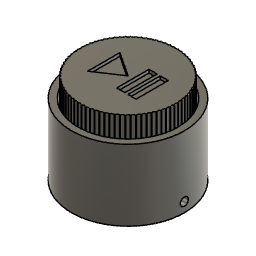
Volume knob v2 (Autodesk Fusion 360 design; units mm, degrees)
Autodesk Fusion 360 part; units mm, degrees
sketch "Sketch1" plane through (0, 0, 0) normal (0, 1, 0) x (1, 0, 0)
  circle A0 centre (0, 0) radius 30
  line L0 (0, 1.6) -> (2.7713, 1.6)
  line L1 (0, 1.6) -> (-2.7713, 1.6)
  arc A1 (-2.7713, 1.6) -> (2.7713, 1.6) centre (0, 0) ccw
  ellipse E0 centre (0, 30) end of major axis (1, 30) minor radius 0.5 (-0.9994, 29.9833) -> (0.9994, 29.9833) ccw
  ellipse E1 centre (-2.3538, 29.9075) end of major axis (-1.3569, 29.986) minor radius 0.5 (-3.3488, 29.8125) -> (-1.3561, 29.9693) ccw
  ellipse E2 centre (-4.693, 29.6307) end of major axis (-3.7053, 29.7871) minor radius 0.5 (-5.6776, 29.4579) -> (-3.7033, 29.7706) ccw
  ellipse E3 centre (-7.0034, 29.1711) end of major axis (-6.031, 29.4045) minor radius 0.5 (-7.9713, 28.9216) -> (-6.0276, 29.3882) ccw
  ellipse E4 centre (-9.2705, 28.5317) end of major axis (-8.3195, 28.8407) minor radius 0.5 (-10.2159, 28.207) -> (-8.3148, 28.8247) ccw
  ellipse E5 centre (-11.4805, 27.7164) end of major axis (-10.5566, 28.0991) minor radius 0.5 (-12.3975, 27.3185) -> (-10.5508, 28.0835) ccw
  ellipse E6 centre (-13.6197, 26.7302) end of major axis (-12.7287, 27.1842) minor radius 0.5 (-14.5027, 26.2616) -> (-12.7216, 27.1691) ccw
  ellipse E7 centre (-15.675, 25.5792) end of major axis (-14.8223, 26.1017) minor radius 0.5 (-16.5184, 25.0428) -> (-14.8141, 26.0872) ccw
  ellipse E8 centre (-17.6336, 24.2705) end of major axis (-16.8245, 24.8583) minor radius 0.5 (-18.4323, 23.6696) -> (-16.8152, 24.8445) ccw
  ellipse E9 centre (-19.4834, 22.8122) end of major axis (-18.723, 23.4616) minor radius 0.5 (-20.2326, 22.1504) -> (-18.7126, 23.4486) ccw
  ellipse E10 centre (-21.2132, 21.2132) end of major axis (-20.5061, 21.9203) minor radius 0.5 (-21.9081, 20.4947) -> (-20.4947, 21.9081) ccw
  ellipse E11 centre (-22.8122, 19.4834) end of major axis (-22.1627, 20.2438) minor radius 0.5 (-23.4486, 18.7126) -> (-22.1504, 20.2326) ccw
  ellipse E12 centre (-24.2705, 17.6336) end of major axis (-23.6827, 18.4426) minor radius 0.5 (-24.8445, 16.8152) -> (-23.6696, 18.4323) ccw
  ellipse E13 centre (-25.5792, 15.675) end of major axis (-25.0567, 16.5276) minor radius 0.5 (-26.0872, 14.8141) -> (-25.0428, 16.5184) ccw
  ellipse E14 centre (-26.7302, 13.6197) end of major axis (-26.2762, 14.5107) minor radius 0.5 (-27.1691, 12.7216) -> (-26.2616, 14.5027) ccw
  ellipse E15 centre (-27.7164, 11.4805) end of major axis (-27.3337, 12.4044) minor radius 0.5 (-28.0835, 10.5508) -> (-27.3185, 12.3975) ccw
  ellipse E16 centre (-28.5317, 9.2705) end of major axis (-28.2227, 10.2216) minor radius 0.5 (-28.8247, 8.3148) -> (-28.207, 10.2159) ccw
  ellipse E17 centre (-29.1711, 7.0034) end of major axis (-28.9377, 7.9757) minor radius 0.5 (-29.3882, 6.0276) -> (-28.9216, 7.9713) ccw
  ellipse E18 centre (-29.6307, 4.693) end of major axis (-29.4742, 5.6807) minor radius 0.5 (-29.7706, 3.7033) -> (-29.4579, 5.6776) ccw
  ellipse E19 centre (-29.9075, 2.3538) end of major axis (-29.8291, 3.3507) minor radius 0.5 (-29.9693, 1.3561) -> (-29.8125, 3.3488) ccw
  ellipse E20 centre (-30, 0) end of major axis (-30, 1) minor radius 0.5 (-29.9833, -0.9994) -> (-29.9833, 0.9994) ccw
  ellipse E21 centre (-29.9075, -2.3538) end of major axis (-29.986, -1.3569) minor radius 0.5 (-29.8125, -3.3488) -> (-29.9693, -1.3561) ccw
  ellipse E22 centre (-29.6307, -4.693) end of major axis (-29.7871, -3.7053) minor radius 0.5 (-29.4579, -5.6776) -> (-29.7706, -3.7033) ccw
  ellipse E23 centre (-29.1711, -7.0034) end of major axis (-29.4045, -6.031) minor radius 0.5 (-28.9216, -7.9713) -> (-29.3882, -6.0276) ccw
  ellipse E24 centre (-28.5317, -9.2705) end of major axis (-28.8407, -8.3195) minor radius 0.5 (-28.207, -10.2159) -> (-28.8247, -8.3148) ccw
  ellipse E25 centre (-27.7164, -11.4805) end of major axis (-28.0991, -10.5566) minor radius 0.5 (-27.3185, -12.3975) -> (-28.0835, -10.5508) ccw
  ellipse E26 centre (-26.7302, -13.6197) end of major axis (-27.1842, -12.7287) minor radius 0.5 (-26.2616, -14.5027) -> (-27.1691, -12.7216) ccw
  ellipse E27 centre (-25.5792, -15.675) end of major axis (-26.1017, -14.8223) minor radius 0.5 (-25.0428, -16.5184) -> (-26.0872, -14.8141) ccw
  ellipse E28 centre (-24.2705, -17.6336) end of major axis (-24.8583, -16.8245) minor radius 0.5 (-23.6696, -18.4323) -> (-24.8445, -16.8152) ccw
  ellipse E29 centre (-22.8122, -19.4834) end of major axis (-23.4616, -18.723) minor radius 0.5 (-22.1504, -20.2326) -> (-23.4486, -18.7126) ccw
  ellipse E30 centre (-21.2132, -21.2132) end of major axis (-21.9203, -20.5061) minor radius 0.5 (-20.4947, -21.9081) -> (-21.9081, -20.4947) ccw
  ellipse E31 centre (-19.4834, -22.8122) end of major axis (-20.2438, -22.1627) minor radius 0.5 (-18.7126, -23.4486) -> (-20.2326, -22.1504) ccw
  ellipse E32 centre (-17.6336, -24.2705) end of major axis (-18.4426, -23.6827) minor radius 0.5 (-16.8152, -24.8445) -> (-18.4323, -23.6696) ccw
  ellipse E33 centre (-15.675, -25.5792) end of major axis (-16.5276, -25.0567) minor radius 0.5 (-14.8141, -26.0872) -> (-16.5184, -25.0428) ccw
  ellipse E34 centre (-13.6197, -26.7302) end of major axis (-14.5107, -26.2762) minor radius 0.5 (-12.7216, -27.1691) -> (-14.5027, -26.2616) ccw
  ellipse E35 centre (-11.4805, -27.7164) end of major axis (-12.4044, -27.3337) minor radius 0.5 (-10.5508, -28.0835) -> (-12.3975, -27.3185) ccw
  ellipse E36 centre (-9.2705, -28.5317) end of major axis (-10.2216, -28.2227) minor radius 0.5 (-8.3148, -28.8247) -> (-10.2159, -28.207) ccw
  ellipse E37 centre (-7.0034, -29.1711) end of major axis (-7.9757, -28.9377) minor radius 0.5 (-6.0276, -29.3882) -> (-7.9713, -28.9216) ccw
  ellipse E38 centre (-4.693, -29.6307) end of major axis (-5.6807, -29.4742) minor radius 0.5 (-3.7033, -29.7706) -> (-5.6776, -29.4579) ccw
  ellipse E39 centre (-2.3538, -29.9075) end of major axis (-3.3507, -29.8291) minor radius 0.5 (-1.3561, -29.9693) -> (-3.3488, -29.8125) ccw
  ellipse E40 centre (0, -30) end of major axis (-1, -30) minor radius 0.5 (0.9994, -29.9833) -> (-0.9994, -29.9833) ccw
  ellipse E41 centre (2.3538, -29.9075) end of major axis (1.3569, -29.986) minor radius 0.5 (3.3488, -29.8125) -> (1.3561, -29.9693) ccw
  ellipse E42 centre (4.693, -29.6307) end of major axis (3.7053, -29.7871) minor radius 0.5 (5.6776, -29.4579) -> (3.7033, -29.7706) ccw
  ellipse E43 centre (7.0034, -29.1711) end of major axis (6.031, -29.4045) minor radius 0.5 (7.9713, -28.9216) -> (6.0276, -29.3882) ccw
  ellipse E44 centre (9.2705, -28.5317) end of major axis (8.3195, -28.8407) minor radius 0.5 (10.2159, -28.207) -> (8.3148, -28.8247) ccw
  ellipse E45 centre (11.4805, -27.7164) end of major axis (10.5566, -28.0991) minor radius 0.5 (12.3975, -27.3185) -> (10.5508, -28.0835) ccw
  ellipse E46 centre (13.6197, -26.7302) end of major axis (12.7287, -27.1842) minor radius 0.5 (14.5027, -26.2616) -> (12.7216, -27.1691) ccw
  ellipse E47 centre (15.675, -25.5792) end of major axis (14.8223, -26.1017) minor radius 0.5 (16.5184, -25.0428) -> (14.8141, -26.0872) ccw
  ellipse E48 centre (17.6336, -24.2705) end of major axis (16.8245, -24.8583) minor radius 0.5 (18.4323, -23.6696) -> (16.8152, -24.8445) ccw
  ellipse E49 centre (19.4834, -22.8122) end of major axis (18.723, -23.4616) minor radius 0.5 (20.2326, -22.1504) -> (18.7126, -23.4486) ccw
  ellipse E50 centre (21.2132, -21.2132) end of major axis (20.5061, -21.9203) minor radius 0.5 (21.9081, -20.4947) -> (20.4947, -21.9081) ccw
  ellipse E51 centre (22.8122, -19.4834) end of major axis (22.1627, -20.2438) minor radius 0.5 (23.4486, -18.7126) -> (22.1504, -20.2326) ccw
  ellipse E52 centre (24.2705, -17.6336) end of major axis (23.6827, -18.4426) minor radius 0.5 (24.8445, -16.8152) -> (23.6696, -18.4323) ccw
  ellipse E53 centre (25.5792, -15.675) end of major axis (25.0567, -16.5276) minor radius 0.5 (26.0872, -14.8141) -> (25.0428, -16.5184) ccw
  ellipse E54 centre (26.7302, -13.6197) end of major axis (26.2762, -14.5107) minor radius 0.5 (27.1691, -12.7216) -> (26.2616, -14.5027) ccw
  ellipse E55 centre (27.7164, -11.4805) end of major axis (27.3337, -12.4044) minor radius 0.5 (28.0835, -10.5508) -> (27.3185, -12.3975) ccw
  ellipse E56 centre (28.5317, -9.2705) end of major axis (28.2227, -10.2216) minor radius 0.5 (28.8247, -8.3148) -> (28.207, -10.2159) ccw
  ellipse E57 centre (29.1711, -7.0034) end of major axis (28.9377, -7.9757) minor radius 0.5 (29.3882, -6.0276) -> (28.9216, -7.9713) ccw
  ellipse E58 centre (29.6307, -4.693) end of major axis (29.4742, -5.6807) minor radius 0.5 (29.7706, -3.7033) -> (29.4579, -5.6776) ccw
  ellipse E59 centre (29.9075, -2.3538) end of major axis (29.8291, -3.3507) minor radius 0.5 (29.9693, -1.3561) -> (29.8125, -3.3488) ccw
  ellipse E60 centre (30, 0) end of major axis (30, -1) minor radius 0.5 (29.9833, 0.9994) -> (29.9833, -0.9994) ccw
  ellipse E61 centre (29.9075, 2.3538) end of major axis (29.986, 1.3569) minor radius 0.5 (29.8125, 3.3488) -> (29.9693, 1.3561) ccw
  ellipse E62 centre (29.6307, 4.693) end of major axis (29.7871, 3.7053) minor radius 0.5 (29.4579, 5.6776) -> (29.7706, 3.7033) ccw
  ellipse E63 centre (29.1711, 7.0034) end of major axis (29.4045, 6.031) minor radius 0.5 (28.9216, 7.9713) -> (29.3882, 6.0276) ccw
  ellipse E64 centre (28.5317, 9.2705) end of major axis (28.8407, 8.3195) minor radius 0.5 (28.207, 10.2159) -> (28.8247, 8.3148) ccw
  ellipse E65 centre (27.7164, 11.4805) end of major axis (28.0991, 10.5566) minor radius 0.5 (27.3185, 12.3975) -> (28.0835, 10.5508) ccw
  ellipse E66 centre (26.7302, 13.6197) end of major axis (27.1842, 12.7287) minor radius 0.5 (26.2616, 14.5027) -> (27.1691, 12.7216) ccw
  ellipse E67 centre (25.5792, 15.675) end of major axis (26.1017, 14.8223) minor radius 0.5 (25.0428, 16.5184) -> (26.0872, 14.8141) ccw
  ellipse E68 centre (24.2705, 17.6336) end of major axis (24.8583, 16.8245) minor radius 0.5 (23.6696, 18.4323) -> (24.8445, 16.8152) ccw
  ellipse E69 centre (22.8122, 19.4834) end of major axis (23.4616, 18.723) minor radius 0.5 (22.1504, 20.2326) -> (23.4486, 18.7126) ccw
  ellipse E70 centre (21.2132, 21.2132) end of major axis (21.9203, 20.5061) minor radius 0.5 (20.4947, 21.9081) -> (21.9081, 20.4947) ccw
  ellipse E71 centre (19.4834, 22.8122) end of major axis (20.2438, 22.1627) minor radius 0.5 (18.7126, 23.4486) -> (20.2326, 22.1504) ccw
  ellipse E72 centre (17.6336, 24.2705) end of major axis (18.4426, 23.6827) minor radius 0.5 (16.8152, 24.8445) -> (18.4323, 23.6696) ccw
  ellipse E73 centre (15.675, 25.5792) end of major axis (16.5276, 25.0567) minor radius 0.5 (14.8141, 26.0872) -> (16.5184, 25.0428) ccw
  ellipse E74 centre (13.6197, 26.7302) end of major axis (14.5107, 26.2762) minor radius 0.5 (12.7216, 27.1691) -> (14.5027, 26.2616) ccw
  ellipse E75 centre (11.4805, 27.7164) end of major axis (12.4044, 27.3337) minor radius 0.5 (10.5508, 28.0835) -> (12.3975, 27.3185) ccw
  ellipse E76 centre (9.2705, 28.5317) end of major axis (10.2216, 28.2227) minor radius 0.5 (8.3148, 28.8247) -> (10.2159, 28.207) ccw
  ellipse E77 centre (7.0034, 29.1711) end of major axis (7.9757, 28.9377) minor radius 0.5 (6.0276, 29.3882) -> (7.9713, 28.9216) ccw
  ellipse E78 centre (4.693, 29.6307) end of major axis (5.6807, 29.4742) minor radius 0.5 (3.7033, 29.7706) -> (5.6776, 29.4579) ccw
  ellipse E79 centre (2.3538, 29.9075) end of major axis (3.3507, 29.8291) minor radius 0.5 (1.3561, 29.9693) -> (3.3488, 29.8125) ccw
  dimension "d1" = 6.4
  dimension "d2" = 60
  dimension "d5" = 360
  constraint coincident A0.centre A1.centre
  constraint coincident A0 E0.centre
  measures "d1" diameter of A1
  measures "d2" diameter of A0
sketch "Sketch2" plane through (0, 0, 0) normal (0, 1, 0) x (1, 0, 0)
  line L0 (-15, 0) -> (-15, 10)
  line L1 (-15, 0) -> (-15, -10)
  line L2 (-15, -10) -> (0, 0)
  line L3 (-15, 10) -> (0, 0)
  line L4 (15, 0) -> (15, 10)
  line L5 (15, 10) -> (10, 10)
  line L6 (10, 10) -> (10, -10)
  line L7 (10, -10) -> (15, -10)
  line L8 (15, -10) -> (15, 0)
  line L9 (8, -10) -> (3, -10)
  line L10 (3, -10) -> (3, 10)
  line L11 (3, 10) -> (8, 10)
  line L12 (8, 10) -> (8, -10)
  constraint coincident L2.end L3.end
  constraint perpendicular L4 L5
  constraint perpendicular L6 L7
  constraint perpendicular L8 L9
  constraint perpendicular L10 L11
  constraint perpendicular L9 L12
extrude "Extrude1" add sketch "Sketch1" along normal blind 25 contours A0 E0 E1 E2 E3 E4 E5 E6 E7 E8 E9 E10 E11 E12 E13 E14 E15 E16 E17 E18 E19 E20 E21 E22 E23 E24 E25 E26 E27 E28 E29 E30 E31 E32 E33 E34 E35 E36 E37 E38 E39 E40 E41 E42 E43 E44 E45 E46 E47 E48 E49 E50 E51 E52 E53 E54 E55 E56 E57 E58 E59 E60 E61 E62 E63 E64 E65 E66 E67 E68 E69 E70 E71 E72 E73 E74 E75 E76 E77 E78 E79 | L0 L1 A1 makes body 1
extrude "Extrude2" cut sketch "Sketch1" along normal blind 15 contours L0 L1 A1 bodies 1
extrude "Extrude3" cut sketch "Sketch2" along normal blind 21 from surface at 23 bodies 1
ref_plane "WorkPlane1" through (0, -6, 0) normal (0, 1, 0) x (0, 0, 1)
sketch "Sketch3" plane through (0, -6, 0) normal (0, 1, 0) x (1, 0, 0)
  circle A0 centre (0, 0) radius 31
  circle A1 centre (0, 0) radius 35
  circle A2 centre (0, 0) radius 3.7
  line L0 (0, 0) -> (0, 10)
  line L1 (0, 0) -> (0, -10)
  line L2 (0, 10) -> (29.3428, 10)
  line L3 (0, -10) -> (29.3428, -10)
  line L4 (0, 10) -> (-29.3428, 10)
  line L5 (0, -10) -> (-29.3428, -10)
  line L6 (-29.3428, 10) -> (-29.3428, -10)
  line L7 (29.3428, -10) -> (29.3428, 10)
  line L8 (0, 29) -> (-10.9545, 29)
  line L9 (0, 29) -> (10.9545, 29)
  line L10 (0, -29) -> (10.9545, -29)
  line L11 (0, -29) -> (-10.9545, -29)
  dimension "d14" = 7.4
  constraint concentric A0 A2
  constraint coincident A0.centre A1.centre
  constraint vertical L1
  constraint coincident A0 L2.end
  constraint perpendicular L0 L2
  constraint coincident A0 L3.end
  constraint perpendicular L1 L3
  constraint perpendicular L0 L4
  constraint perpendicular L1 L5
  constraint coincident A0 L4.end
  constraint coincident A0 L5.end
  constraint perpendicular L5 L6
  constraint coincident A0 L11.end
  constraint coincident A0 L10.end
  constraint coincident A0 L9.end
  constraint coincident A0 L8.end
  measures "d14" diameter of A2
extrude "Extrude4" add sketch "Sketch3" against normal blind 4 separate body contours A0 L7 | A0 L2 L4 L8 L9 | A2 L0 L1 L2 L3 L7 | A0 L3 L5 L10 L11 | A0 L8 L9 | A2 L0 L1 L4 L5 L6 | A0 L10 L11 | A0 L6 makes body 2
extrude "Extrude5" add sketch "Sketch3" along normal blind 10 and the other way blind 34 separate body makes body 3
extrude "Extrude6" add sketch "Sketch3" against normal blind 29.9 from surface at -4.1 contours A0 L7 | A0 L8 L9 | A0 L10 L11 | A0 L6 bodies 3
extrude "Extrude7" add sketch "Sketch3" along normal blind 3 from surface at -34 contours A2 L0 L1 L2 L3 L7 | A2 L0 L1 L4 L5 L6 bodies 3
sketch "Sketch4" plane through (29.3428, 0, 0) normal (-1, 0, 0) x (0, 0, 1)
  line L0 (-10, -37) -> (10, -37)
  line L1 (10, -37) -> (10, -10.1)
  line L2 (10, -10.1) -> (-10, -10.1)
  line L3 (-10, -10.1) -> (-10, -37)
  circle A0 centre (0, -34) radius 2.5
  dimension "d27" = 5
  measures "d27" diameter of A0
extrude "Extrude8" cut sketch "Sketch4" against normal blind 13 contours A0 bodies 3
ref_plane "WorkPlane2" through (0, 22, 0) normal (0, 1, 0) x (1, 0, 0)
ref_plane "WorkPlane3" through (0, 13, 0) normal (0, 1, 0) x (1, 0, 0)
split "Split1" by plane through (0, 13, 0) normal (0, 1, 0) and through (0, 22, 0) normal (0, 1, 0) bodies 1 makes body 4 at (-7.0247, 25, 16.0234) makes body 5 at (-2.9168, 13.6667, -1.3161)
combine "Combine1" operation add target body 4 tool bodies 1 makes body 6 at (0.0045, 13, -10.9)
move_body "Move1" bodies 4 to x (1, 0, 0) y (0, 1, 0) z (0, 0, 1) at (0, -9, 0)
combine "Combine2" operation add target body 6 tool bodies 4
hidden bodies 5
